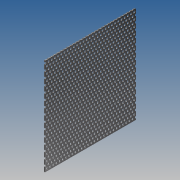
# Autodesk Inventor part: DD_KVD_003_07
Saved by Autodesk Inventor 2017.3 (Build 213256000, 256)
## iProperties
Created: 2023-12-04
Part Number: DD_KVD_003_07
Material: Nerezová ocel
Document SubType Name: Sheet Metal
Designer: Darena
Density: 8 g/cm^3
Flat Pattern Width: 27.5 cm
Flat Pattern Length: 25.8 cm
Flat Pattern Area: 709.5 cm^2
Sheet Metal Rule: Výchozí_mm
Sheet Metal Width: 275,000 mm
Sheet Metal Length: 258,000 mm
Sheet Metal Area: 70950,000 mm^2
Appearance: Pololeštěná
Author: Darena
Title: DÍL SVAŘENCE - 13
Autodesk Inventor part; units mm, degrees
ref_plane "YZ Plane" through (0, 0, 0) normal (1, 0, 0) x (0, 1, 0)
ref_plane "XZ Plane" through (0, 0, 0) normal (0, 1, 0) x (-1, 0, 0)
ref_plane "XY Plane" through (0, 0, 0) normal (0, 0, 1) x (1, 0, 0)
sketch "Náčrt2" plane through (0, 0, 0) normal (1, 0, 0) x (0, 1, 0)
  line L0 (129, 137.5) -> (-129, 137.5)
  line L1 (-129, 137.5) -> (-129, -137.5)
  line L2 (-129, -137.5) -> (129, -137.5)
  line L3 (129, -137.5) -> (129, 137.5)
  point P0 (0, 0)
  point P1 (-129, 0)
  point P2 (0, 137.5)
  dimension "d0" = 275
  dimension "d1" = 258
  constraints: 8 end point, 2 midpoint, 2 parallel, 1 horizontal, 1 horizontal alignment, 1 perpendicular, 1 vertical alignment
  measures "d0" distance of L0.end L1.end
  measures "d1" distance of L0.start L0.end
extrude "Vysunutí1" add sketch "Náčrt2" against normal blind 2.5
sketch "Náčrt9" plane through (0, 0, 0) normal (1, 0, 0) x (0, 0, -1)
  circle A0 centre (-139.1359, -122.8641) radius 3
  line L0 (-137.5, -129) -> (137.5, -129) projected
  circle A1 centre (-130.1359, -118.3641) radius 3
  circle A2 centre (-130.1359, -127.3641) radius 3
  line L1 (-130.1359, -127.3641) -> (-130.1359, -118.3641) construction
  line L2 (-139.1359, -122.8641) -> (-130.1359, -122.8641) construction
  circle A3 centre (-139.1359, -131.8641) radius 3 construction
  line L3 (-137.5, 129) -> (-137.5, -129) projected
  line L4 (-139.1359, -131.8641) -> (-139.1359, -122.8641) construction
  circle A4 centre (-121.1359, -122.8641) radius 3
  line L5 (-130.1359, -122.8641) -> (-121.1359, -122.8641) construction
  point P0 (0, 0)
  dimension "d45" = 6
  dimension "d52" = 9
  dimension "d56" = 1.6359
  dimension "d57" = 1.6359
  constraints: 8 end point, 5 centre point, 4 equal radius, 3 equal length, 2 vertical, 1 collinear, 1 midpoint, 1 perpendicular
  measures "d45" diameter of A0
  measures "d52" distance of L1.end L1.start
  measures "d56" distance between parallel lines of L3 L4
  measures "d57" distance from line of L0 L1.start
extrude "Vysunutí5" cut sketch "Náčrt9" against normal through all
pattern_linear "Obdélníkové pole1" count 15 spacing 18 along (0, 0, -1) count 29 spacing 9 along (0, 1, 0) of "Vysunutí5"
equation "\"d57\" = d56"
equation "\"PoloměrOhybu\" = Tloušťka"
equation "\"ŠířkaVýštipu\" = Tloušťka"
equation "\"HloubkaVýštipu\" = 0.5 * Tloušťka"
equation "\"MinimálníZbytek\" = 2 * Tloušťka"
equation "\"PřechodovýPoloměr\" = PoloměrOhybu"
equation "\"VelikostJacobihoPoloměru\" = PoloměrOhybu"
equation "\"VelikostMezery\" = Tloušťka"
equation "\"Tloušťka\" = 2.5"
